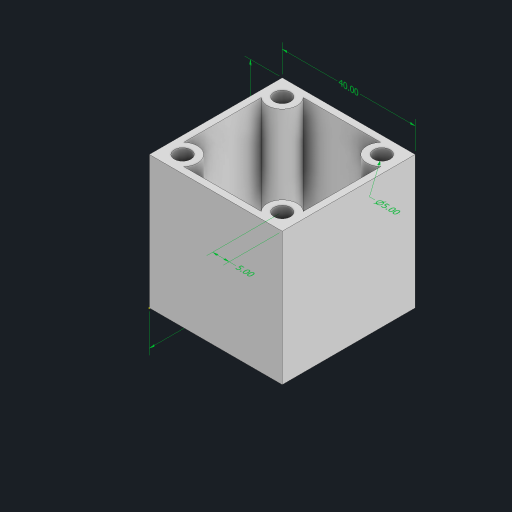
# Autodesk Inventor part: INTRO_CUBE
Saved by Autodesk Inventor 2023 (Build 270158000, 158)
## iProperties
Created: 2023-03-07
Part Number: INTRO_CUBE
Material: Generic
Document SubType Name: Modeling
Designer: n9379410
Density: 1 g/cm^3
Appearance: Default
Author: n9379410
Autodesk Inventor part; units mm, degrees
ref_plane "YZ Plane" through (0, 0, 0) normal (1, 0, 0) x (0, 1, 0)
ref_plane "XZ Plane" through (0, 0, 0) normal (0, 1, 0) x (-1, 0, 0)
ref_plane "XY Plane" through (0, 0, 0) normal (0, 0, 1) x (1, 0, 0)
sketch "cube_profile" plane through (0, 0, 0) normal (0, 1, 0) x (-1, 0, 0)
  line L0 (0, 0) -> (-40, 0)
  line L1 (-40, 0) -> (-40, -40)
  line L2 (-40, -40) -> (0, -40)
  line L3 (0, -40) -> (0, 0)
  dimension "d2" = 40
  dimension "d4" = 40
  constraints: 8 end point, 2 parallel, 1 coincident, 1 horizontal, 1 perpendicular
  measures "d2" distance of L0.end L1.end
  measures "d4" distance of L1.end L2.end
extrude "Extrusion1" add sketch "cube_profile" along normal blind 40
sketch "Sketch2" plane through (0, 40, 0) normal (0, 1, 0) x (1, 0, 0)
  line L0 (40, 40) -> (0, 40) projected
  line L1 (0, 40) -> (0, 0) projected
  circle A0 centre (5, 35) radius 2.5
  circle A1 centre (35, 35) radius 2.5
  circle A2 centre (5, 5) radius 2.5
  circle A3 centre (35, 5) radius 2.5
  dimension "d8" = 5
  dimension "d9" = 5
  dimension "d10" = 5
  dimension "d13" = 30
  dimension "d16" = 30
  constraints: 4 centre point, 1 coincident, 1 horizontal, 1 vertical, 6 other
  measures "d8" distance from line of L0 point (5, 35)
  measures "d9" distance from line of L1 point (5, 35)
  measures "d10" diameter of A0
  measures "d13" distance of A0.centre A1.centre
  measures "d16" distance of A0.centre A2.centre
extrude "Extrusion2" cut sketch "Sketch2" against normal blind 50.325
shell "Shell1" thickness 2 removed faces 1 at (24.3762, 40, -24.4474)
sketch "Sketch3" plane through (0, 0, 0) normal (0, 0, 1) x (1, 0, 0)
  point P0 (0, 0)
body "Solid1"
